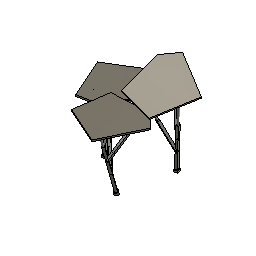
TT-3 (Autodesk Fusion 360 design; units mm, degrees)
Autodesk Fusion 360 part; units mm, degrees
sketch "Sketch1" plane through (0, 0, 0) normal (0, 1, 0) x (1, 0, 0) in component "TT-2 v5"
  line L0 (2.5, -2.5) -> (-2.5, -2.5)
  line L1 (-2.5, -2.5) -> (-2.5, 2.5)
  line L2 (-2.5, 2.5) -> (2.5, 2.5)
  line L3 (2.5, 2.5) -> (2.5, -2.5)
  constraint horizontal L0
  constraint vertical L1
  constraint horizontal L2
  constraint vertical L3
extrude "Extrude1" add sketch "Sketch1" along normal blind 2.5 makes body 1 in component "TT-2 v5"
sketch "Sketch2" plane through (0, 0, 0) normal (0, 1, 0) x (1, 0, 0) in component "TT-2 v5"
  line L0 (1.5, -1.5) -> (-1.5, -1.5)
  line L1 (-1.5, -1.5) -> (-1.5, 1.5)
  line L2 (-1.5, 1.5) -> (1.5, 1.5)
  line L3 (1.5, 1.5) -> (1.5, -1.5)
  constraint horizontal L0
  constraint vertical L1
  constraint horizontal L2
  constraint vertical L3
extrude "Extrude2" add sketch "Sketch2" along normal blind 60 separate body makes body 2 in component "TT-2 v5"
move_body "Move1" bodies 2 to x (0.939693, -0.34202, 0) y (0.34202, 0.939693, 0) z (0, 0, 1) at (-0.0905, -0.513, 0) in component "TT-2 v5"
move_body "Move2" bodies 2 to x (1, 0, 0) y (0, 1, 0) z (0, 0, 1) at (3.3727, 9.6612, 0) in component "TT-2 v5"
sphere "SpherePrimitive1" add diameter 3 placed x (0, 0, 1) y (-0.939693, 0.34202, 0) z (-0.34202, -0.939693, 0) at (3.3241, 9.1329, 0) bodies 2 in component "TT-2 v5"
sphere "SpherePrimitive2" cut diameter 3 placed x (-1, 0, 0) y (0, 0, 1) z (0, 1, 0) at (0, 2.5, 0) bodies 1 in component "TT-2 v5"
cylinder "CylinderPrimitive1" add diameter 2.5 height 40 placed x (0.883022, -0.321394, -0.34202) y (-0.321394, 0.116978, -0.939693) z (0.34202, 0.939693, 0) at (23.8453, 65.5145, 0) separate body makes body 3 in component "TT-2 v5"
sphere "SpherePrimitive3" add diameter 2.5 placed x (0, 0, -1) y (-0.939693, 0.34202, 0) z (0.34202, 0.939693, 0) at (37.5261, 103.1022, 0) bodies 3 in component "TT-2 v5"
move_body "Move3" bodies 3 2 to x (0.939693, 0.34202, 0) y (-0.34202, 0.939693, 0) z (0, 0, 1) at (23.6283, -3.8286, 0) in component "TT-2 v5"
move_body "Move4" bodies 2 3 to x (1, 0, 0) y (0, 1, 0) z (0, 0, 1) at (-23.6681, -3.196, 0) in component "TT-2 v5"
copy_body "CopyPasteBodies1" bodies 3 2 makes body 4 makes body 5 in component "TT-2 v5"
move_body "Move5" bodies 4 5 to x (1, 0, 0) y (0, 0.906308, 0.422618) z (0, -0.422618, 0.906308) at (0, 42.015, -10.6133) in component "TT-2 v5"
move_body "Move6" bodies 5 4 to x (1, 0, 0) y (0, 1, 0) z (0, 0, 1) at (0, -2.8403, 9.6134) in component "TT-2 v5"
extrude "Extrude3" cut 1 faces at (0.4157, 96.2065, 25.0427) along direction (0, -0.906308, -0.422618) blind 15 on bodies 5 bodies 5 in component "TT-2 v5"
move_body "Move7" bodies 4 to x (1, 0, 0) y (0, 1, 0) z (0, 0, 1) at (0, -26.7116, -12.4558) in component "TT-2 v5"
move_body "Move8" bodies 5 4 to x (1, 0, 0) y (0, 1, 0) z (0, 0, 1) at (0, -15.5908, 0) in component "TT-2 v5"
copy_body "CopyPasteBodies2" bodies 4 5 makes body 6 makes body 7 in component "TT-2 v5"
move_body "Move9" bodies 6 7 to x (0, 0, -1) y (0, 1, 0) z (1, 0, 0) at (-0.0791, 0, -0.06) in component "TT-2 v5"
move_body "Move10" bodies 6 to x (1, 0, 0) y (0, 1, 0) z (0, 0, 1) at (5.2397, 11.2365, 0) in component "TT-2 v5"
move_body "Move11" bodies 7 3 4 2 5 6 to x (1, 0, 0) y (0, 0.984808, -0.173648) z (0, 0.173648, 0.984808) at (0, 0.0409, 0.4679) in component "TT-2 v5"
move_body "Move12" bodies 5 4 to x (1, 0, 0) y (0, 1, 0) z (0, 0, 1) at (0, 17.3834, -3.0131) in component "TT-2 v5"
sketch "Sketch7" plane through (0, 0, 0) normal (0, 1, 0) x (1, 0, 0) in component "TT-2 v5"
  line L0 (20, -30) -> (50, 15)
  line L1 (50, 15) -> (20, 47.2574)
  line L2 (20, 47.2574) -> (-26.886, 18.4817)
  line L3 (-26.886, 18.4817) -> (-3.443, -34.2088)
  line L4 (-3.443, -34.2088) -> (20, -30)
extrude "Extrude4" add sketch "Sketch7" along normal blind 2 separate body makes body 8 in component "TT-2 v5"
move_body "Move13" bodies 8 to x (1, 0, 0) y (0, 1, 0) z (0, 0, 1) at (0, 114.7446, 0) in component "TT-2 v5"
sketch "Sketch8" plane through (0, 114.7446, 0) normal (0, -1, 0) x (1, 0, 0) in component "TT-2 v5"
  line L0 (20, 30) -> (-3.443, 34.2088)
  line L1 (-3.443, 34.2088) -> (-26.886, -18.4817)
  line L2 (-26.886, -18.4817) -> (20, -47.2574)
  line L3 (20, -47.2574) -> (50, -15)
  line L4 (50, -15) -> (20, 30)
sphere "SpherePrimitive4" cut diameter 2.5 placed x (1, 0, 0) y (0, 0, 1) z (0, -1, 0) at (-5, 114.7446, -17) bodies 8 in component "TT-2 v5"
sphere "SpherePrimitive5" cut diameter 2.5 placed x (1, 0, 0) y (0, 0, 1) z (0, -1, 0) at (3, 114.7446, 17) bodies 8 in component "TT-2 v5"
sphere "SpherePrimitive6" cut diameter 2.5 placed x (1, 0, 0) y (0, 0, 1) z (0, -1, 0) at (32.239, 114.7446, -14.3242) bodies 8 in component "TT-2 v5"
copy_body "CopyPasteBodies3" bodies 7 5 makes body 9 makes body 10 in component "TT-2 v5"
extrude "Extrude5" cut 1 faces at (19.5306, 65.7186, -10.5804) along direction (-0.422618, -0.892539, 0.157379) blind 45 on bodies 9 bodies 9 in component "TT-2 v5"
extrude "Extrude6" cut 1 faces at (-0.5843, 86.4162, 5.2019) along direction (0, -0.965926, -0.258819) blind 45 on bodies 10 bodies 10 in component "TT-2 v5"
combine "Combine1" operation cut target body 2 tool bodies 9 in component "TT-2 v5"
combine "Combine2" operation cut target body 2 tool bodies 10 in component "TT-2 v5"
copy_body "CopyPasteBodies4" bodies 7 5 makes body 11 makes body 12 in component "TT-2 v5"
combine "Combine3" operation cut target body 2 tool bodies 11 12 in component "TT-2 v5"
copy_body "Body->Comp1" bodies 1 removing the originals makes body 13 in component "MainFix"
copy_body "Body->Comp2" bodies 3 removing the originals makes body 14 in component "MainAct"
copy_body "Body->Comp3" bodies 4 removing the originals makes body 15 in component "LeftAct"
copy_body "Body->Comp4" bodies 2 removing the originals makes body 16 in component "MainBranch"
copy_body "Body->Comp5" bodies 5 removing the originals makes body 17 in component "LeftBranch"
copy_body "Body->Comp6" bodies 6 removing the originals makes body 18 in component "RightAct"
copy_body "Body->Comp7" bodies 7 removing the originals makes body 19 in component "RightBranch"
copy_body "Body->Comp8" bodies 8 removing the originals makes body 20 in component "Flat"
sketch "Sketch1 (2)" plane through (0, 0, 0) normal (0, 1, 0) x (1, 0, 0) in component "TT-2 v5 (1)"
  line L0 (2.5, -2.5) -> (-2.5, -2.5)
  line L1 (-2.5, -2.5) -> (-2.5, 2.5)
  line L2 (-2.5, 2.5) -> (2.5, 2.5)
  line L3 (2.5, 2.5) -> (2.5, -2.5)
  constraint horizontal L0
  constraint vertical L1
  constraint horizontal L2
  constraint vertical L3
extrude "Extrude1'" add sketch "Sketch1 (2)" along normal blind 2.5 separate body makes body 21 in component "TT-2 v5 (1)"
sketch "Sketch2 (2)" plane through (0, 0, 0) normal (0, 1, 0) x (1, 0, 0) in component "TT-2 v5 (1)"
  line L0 (1.5, -1.5) -> (-1.5, -1.5)
  line L1 (-1.5, -1.5) -> (-1.5, 1.5)
  line L2 (-1.5, 1.5) -> (1.5, 1.5)
  line L3 (1.5, 1.5) -> (1.5, -1.5)
  constraint horizontal L0
  constraint vertical L1
  constraint horizontal L2
  constraint vertical L3
extrude "Extrude2'" add sketch "Sketch2 (2)" along normal blind 60 separate body makes body 22 in component "TT-2 v5 (1)"
move_body "Move1'" bodies 22 to x (0.939693, -0.34202, 0) y (0.34202, 0.939693, 0) z (0, 0, 1) at (-0.0905, -0.513, 0) in component "TT-2 v5 (1)"
move_body "Move2'" bodies 22 to x (1, 0, 0) y (0, 1, 0) z (0, 0, 1) at (3.3727, 9.6612, 0) in component "TT-2 v5 (1)"
sphere "SpherePrimitive1'" add diameter 3 placed x (0, 0, 1) y (-0.939693, 0.34202, 0) z (-0.34202, -0.939693, 0) at (3.3241, 9.1329, 0) bodies 22 in component "TT-2 v5 (1)"
sphere "SpherePrimitive2'" cut diameter 3 placed x (-1, 0, 0) y (0, 0, 1) z (0, 1, 0) at (0, 2.5, 0) bodies 21 in component "TT-2 v5 (1)"
cylinder "CylinderPrimitive1'" add diameter 2.5 height 40 placed x (0.883022, -0.321394, -0.34202) y (-0.321394, 0.116978, -0.939693) z (0.34202, 0.939693, 0) at (23.8453, 65.5145, 0) separate body makes body 23 in component "TT-2 v5 (1)"
sphere "SpherePrimitive3'" add diameter 2.5 placed x (0, 0, -1) y (-0.939693, 0.34202, 0) z (0.34202, 0.939693, 0) at (37.5261, 103.1022, 0) bodies 23 in component "TT-2 v5 (1)"
move_body "Move3'" bodies 23 22 to x (0.939693, 0.34202, 0) y (-0.34202, 0.939693, 0) z (0, 0, 1) at (23.6283, -3.8286, 0) in component "TT-2 v5 (1)"
move_body "Move4'" bodies 22 23 to x (1, 0, 0) y (0, 1, 0) z (0, 0, 1) at (-23.6681, -3.196, 0) in component "TT-2 v5 (1)"
copy_body "CopyPasteBodies1'" bodies 23 22 makes body 24 makes body 25 in component "TT-2 v5 (1)"
move_body "Move5'" bodies 24 25 to x (1, 0, 0) y (0, 0.906308, 0.422618) z (0, -0.422618, 0.906308) at (0, 42.015, -10.6133) in component "TT-2 v5 (1)"
move_body "Move6'" bodies 25 24 to x (1, 0, 0) y (0, 1, 0) z (0, 0, 1) at (0, -2.8403, 9.6134) in component "TT-2 v5 (1)"
extrude "Extrude3'" cut 1 faces at (0.4157, 96.2065, 25.0427) along direction (0, -0.906308, -0.422618) blind 15 on bodies 25 bodies 25 in component "TT-2 v5 (1)"
move_body "Move7'" bodies 24 to x (1, 0, 0) y (0, 1, 0) z (0, 0, 1) at (0, -26.7116, -12.4558) in component "TT-2 v5 (1)"
move_body "Move8'" bodies 25 24 to x (1, 0, 0) y (0, 1, 0) z (0, 0, 1) at (0, -15.5908, 0) in component "TT-2 v5 (1)"
copy_body "CopyPasteBodies2'" bodies 24 25 makes body 26 makes body 27 in component "TT-2 v5 (1)"
move_body "Move9'" bodies 26 27 to x (0, 0, -1) y (0, 1, 0) z (1, 0, 0) at (-0.0791, 0, -0.06) in component "TT-2 v5 (1)"
move_body "Move10'" bodies 26 to x (1, 0, 0) y (0, 1, 0) z (0, 0, 1) at (5.2397, 11.2365, 0) in component "TT-2 v5 (1)"
move_body "Move11'" bodies 27 23 24 22 25 26 to x (1, 0, 0) y (0, 0.984808, -0.173648) z (0, 0.173648, 0.984808) at (0, 0.0409, 0.4679) in component "TT-2 v5 (1)"
move_body "Move12'" bodies 25 24 to x (1, 0, 0) y (0, 1, 0) z (0, 0, 1) at (0, 17.3834, -3.0131) in component "TT-2 v5 (1)"
sketch "Sketch7 (2)" plane through (0, 0, 0) normal (0, 1, 0) x (1, 0, 0) in component "TT-2 v5 (1)"
  line L0 (20, -30) -> (50, 15)
  line L1 (50, 15) -> (20, 47.2574)
  line L2 (20, 47.2574) -> (-26.886, 18.4817)
  line L3 (-26.886, 18.4817) -> (-3.443, -34.2088)
  line L4 (-3.443, -34.2088) -> (20, -30)
extrude "Extrude4'" add sketch "Sketch7 (2)" along normal blind 2 separate body makes body 28 in component "TT-2 v5 (1)"
move_body "Move13'" bodies 28 to x (1, 0, 0) y (0, 1, 0) z (0, 0, 1) at (0, 114.7446, 0) in component "TT-2 v5 (1)"
sketch "Sketch8 (2)" plane through (0, 114.7446, 0) normal (0, -1, 0) x (1, 0, 0) in component "TT-2 v5 (1)"
  line L0 (20, 30) -> (-3.443, 34.2088)
  line L1 (-3.443, 34.2088) -> (-26.886, -18.4817)
  line L2 (-26.886, -18.4817) -> (20, -47.2574)
  line L3 (20, -47.2574) -> (50, -15)
  line L4 (50, -15) -> (20, 30)
sphere "SpherePrimitive4'" cut diameter 2.5 placed x (1, 0, 0) y (0, 0, 1) z (0, -1, 0) at (-5, 114.7446, -17) bodies 28 in component "TT-2 v5 (1)"
sphere "SpherePrimitive5'" cut diameter 2.5 placed x (1, 0, 0) y (0, 0, 1) z (0, -1, 0) at (3, 114.7446, 17) bodies 28 in component "TT-2 v5 (1)"
sphere "SpherePrimitive6'" cut diameter 2.5 placed x (1, 0, 0) y (0, 0, 1) z (0, -1, 0) at (32.239, 114.7446, -14.3242) bodies 28 in component "TT-2 v5 (1)"
copy_body "CopyPasteBodies3'" bodies 27 25 makes body 29 makes body 30 in component "TT-2 v5 (1)"
extrude "Extrude5'" cut 1 faces at (19.5306, 65.7186, -10.5804) along direction (-0.422618, -0.892539, 0.157379) blind 45 on bodies 29 bodies 29 in component "TT-2 v5 (1)"
extrude "Extrude6'" cut 1 faces at (-0.5843, 86.4162, 5.2019) along direction (0, -0.965926, -0.258819) blind 45 on bodies 30 bodies 30 in component "TT-2 v5 (1)"
combine "Combine1'" operation cut target body 22 tool bodies 29 in component "TT-2 v5 (1)"
combine "Combine2'" operation cut target body 22 tool bodies 30 in component "TT-2 v5 (1)"
copy_body "CopyPasteBodies4'" bodies 27 25 makes body 31 makes body 32 in component "TT-2 v5 (1)"
combine "Combine3'" operation cut target body 22 tool bodies 31 32 in component "TT-2 v5 (1)"
copy_body "Body->Comp1'" bodies 21 removing the originals makes body 33 in component "MainFix (1)"
copy_body "Body->Comp2'" bodies 23 removing the originals makes body 34 in component "MainAct (1)"
copy_body "Body->Comp3'" bodies 24 removing the originals makes body 35 in component "LeftAct (1)"
copy_body "Body->Comp4'" bodies 22 removing the originals makes body 36 in component "MainBranch (1)"
copy_body "Body->Comp5'" bodies 25 removing the originals makes body 37 in component "LeftBranch (1)"
copy_body "Body->Comp6'" bodies 26 removing the originals makes body 38 in component "RightAct (1)"
copy_body "Body->Comp7'" bodies 27 removing the originals makes body 39 in component "RightBranch (1)"
copy_body "Body->Comp8'" bodies 28 removing the originals makes body 40 in component "Flat (1)"
sketch "Sketch1 (3)" plane through (0, 0, 0) normal (0, 1, 0) x (1, 0, 0) in component "TT-2 v5 (2)"
  line L0 (2.5, -2.5) -> (-2.5, -2.5)
  line L1 (-2.5, -2.5) -> (-2.5, 2.5)
  line L2 (-2.5, 2.5) -> (2.5, 2.5)
  line L3 (2.5, 2.5) -> (2.5, -2.5)
  constraint horizontal L0
  constraint vertical L1
  constraint horizontal L2
  constraint vertical L3
extrude "Extrude1''" add sketch "Sketch1 (3)" along normal blind 2.5 separate body makes body 41 in component "TT-2 v5 (2)"
sketch "Sketch2 (3)" plane through (0, 0, 0) normal (0, 1, 0) x (1, 0, 0) in component "TT-2 v5 (2)"
  line L0 (1.5, -1.5) -> (-1.5, -1.5)
  line L1 (-1.5, -1.5) -> (-1.5, 1.5)
  line L2 (-1.5, 1.5) -> (1.5, 1.5)
  line L3 (1.5, 1.5) -> (1.5, -1.5)
  constraint horizontal L0
  constraint vertical L1
  constraint horizontal L2
  constraint vertical L3
extrude "Extrude2''" add sketch "Sketch2 (3)" along normal blind 60 separate body makes body 42 in component "TT-2 v5 (2)"
move_body "Move1''" bodies 42 to x (0.939693, -0.34202, 0) y (0.34202, 0.939693, 0) z (0, 0, 1) at (-0.0905, -0.513, 0) in component "TT-2 v5 (2)"
move_body "Move2''" bodies 42 to x (1, 0, 0) y (0, 1, 0) z (0, 0, 1) at (3.3727, 9.6612, 0) in component "TT-2 v5 (2)"
sphere "SpherePrimitive1''" add diameter 3 placed x (0, 0, 1) y (-0.939693, 0.34202, 0) z (-0.34202, -0.939693, 0) at (3.3241, 9.1329, 0) bodies 42 in component "TT-2 v5 (2)"
sphere "SpherePrimitive2''" cut diameter 3 placed x (-1, 0, 0) y (0, 0, 1) z (0, 1, 0) at (0, 2.5, 0) bodies 41 in component "TT-2 v5 (2)"
cylinder "CylinderPrimitive1''" add diameter 2.5 height 40 placed x (0.883022, -0.321394, -0.34202) y (-0.321394, 0.116978, -0.939693) z (0.34202, 0.939693, 0) at (23.8453, 65.5145, 0) separate body makes body 43 in component "TT-2 v5 (2)"
sphere "SpherePrimitive3''" add diameter 2.5 placed x (0, 0, -1) y (-0.939693, 0.34202, 0) z (0.34202, 0.939693, 0) at (37.5261, 103.1022, 0) bodies 43 in component "TT-2 v5 (2)"
move_body "Move3''" bodies 43 42 to x (0.939693, 0.34202, 0) y (-0.34202, 0.939693, 0) z (0, 0, 1) at (23.6283, -3.8286, 0) in component "TT-2 v5 (2)"
move_body "Move4''" bodies 42 43 to x (1, 0, 0) y (0, 1, 0) z (0, 0, 1) at (-23.6681, -3.196, 0) in component "TT-2 v5 (2)"
copy_body "CopyPasteBodies1''" bodies 43 42 makes body 44 makes body 45 in component "TT-2 v5 (2)"
move_body "Move5''" bodies 44 45 to x (1, 0, 0) y (0, 0.906308, 0.422618) z (0, -0.422618, 0.906308) at (0, 42.015, -10.6133) in component "TT-2 v5 (2)"
move_body "Move6''" bodies 45 44 to x (1, 0, 0) y (0, 1, 0) z (0, 0, 1) at (0, -2.8403, 9.6134) in component "TT-2 v5 (2)"
extrude "Extrude3''" cut 1 faces at (0.4157, 96.2065, 25.0427) along direction (0, -0.906308, -0.422618) blind 15 on bodies 45 bodies 45 in component "TT-2 v5 (2)"
move_body "Move7''" bodies 44 to x (1, 0, 0) y (0, 1, 0) z (0, 0, 1) at (0, -26.7116, -12.4558) in component "TT-2 v5 (2)"
move_body "Move8''" bodies 45 44 to x (1, 0, 0) y (0, 1, 0) z (0, 0, 1) at (0, -15.5908, 0) in component "TT-2 v5 (2)"
copy_body "CopyPasteBodies2''" bodies 44 45 makes body 46 makes body 47 in component "TT-2 v5 (2)"
move_body "Move9''" bodies 46 47 to x (0, 0, -1) y (0, 1, 0) z (1, 0, 0) at (-0.0791, 0, -0.06) in component "TT-2 v5 (2)"
move_body "Move10''" bodies 46 to x (1, 0, 0) y (0, 1, 0) z (0, 0, 1) at (5.2397, 11.2365, 0) in component "TT-2 v5 (2)"
move_body "Move11''" bodies 47 43 44 42 45 46 to x (1, 0, 0) y (0, 0.984808, -0.173648) z (0, 0.173648, 0.984808) at (0, 0.0409, 0.4679) in component "TT-2 v5 (2)"
move_body "Move12''" bodies 45 44 to x (1, 0, 0) y (0, 1, 0) z (0, 0, 1) at (0, 17.3834, -3.0131) in component "TT-2 v5 (2)"
sketch "Sketch7 (3)" plane through (0, 0, 0) normal (0, 1, 0) x (1, 0, 0) in component "TT-2 v5 (2)"
  line L0 (20, -30) -> (50, 15)
  line L1 (50, 15) -> (20, 47.2574)
  line L2 (20, 47.2574) -> (-26.886, 18.4817)
  line L3 (-26.886, 18.4817) -> (-3.443, -34.2088)
  line L4 (-3.443, -34.2088) -> (20, -30)
extrude "Extrude4''" add sketch "Sketch7 (3)" along normal blind 2 separate body makes body 48 in component "TT-2 v5 (2)"
move_body "Move13''" bodies 48 to x (1, 0, 0) y (0, 1, 0) z (0, 0, 1) at (0, 114.7446, 0) in component "TT-2 v5 (2)"
sketch "Sketch8 (3)" plane through (0, 114.7446, 0) normal (0, -1, 0) x (1, 0, 0) in component "TT-2 v5 (2)"
  line L0 (20, 30) -> (-3.443, 34.2088)
  line L1 (-3.443, 34.2088) -> (-26.886, -18.4817)
  line L2 (-26.886, -18.4817) -> (20, -47.2574)
  line L3 (20, -47.2574) -> (50, -15)
  line L4 (50, -15) -> (20, 30)
sphere "SpherePrimitive4''" cut diameter 2.5 placed x (1, 0, 0) y (0, 0, 1) z (0, -1, 0) at (-5, 114.7446, -17) bodies 48 in component "TT-2 v5 (2)"
sphere "SpherePrimitive5''" cut diameter 2.5 placed x (1, 0, 0) y (0, 0, 1) z (0, -1, 0) at (3, 114.7446, 17) bodies 48 in component "TT-2 v5 (2)"
sphere "SpherePrimitive6''" cut diameter 2.5 placed x (1, 0, 0) y (0, 0, 1) z (0, -1, 0) at (32.239, 114.7446, -14.3242) bodies 48 in component "TT-2 v5 (2)"
copy_body "CopyPasteBodies3''" bodies 47 45 makes body 49 makes body 50 in component "TT-2 v5 (2)"
extrude "Extrude5''" cut 1 faces at (19.5306, 65.7186, -10.5804) along direction (-0.422618, -0.892539, 0.157379) blind 45 on bodies 49 bodies 49 in component "TT-2 v5 (2)"
extrude "Extrude6''" cut 1 faces at (-0.5843, 86.4162, 5.2019) along direction (0, -0.965926, -0.258819) blind 45 on bodies 50 bodies 50 in component "TT-2 v5 (2)"
combine "Combine1''" operation cut target body 42 tool bodies 49 in component "TT-2 v5 (2)"
combine "Combine2''" operation cut target body 42 tool bodies 50 in component "TT-2 v5 (2)"
copy_body "CopyPasteBodies4''" bodies 47 45 makes body 51 makes body 52 in component "TT-2 v5 (2)"
combine "Combine3''" operation cut target body 42 tool bodies 51 52 in component "TT-2 v5 (2)"
copy_body "Body->Comp1''" bodies 41 removing the originals makes body 53 in component "MainFix (2)"
copy_body "Body->Comp2''" bodies 43 removing the originals makes body 54 in component "MainAct (2)"
copy_body "Body->Comp3''" bodies 44 removing the originals makes body 55 in component "LeftAct (2)"
copy_body "Body->Comp4''" bodies 42 removing the originals makes body 56 in component "MainBranch (2)"
copy_body "Body->Comp5''" bodies 45 removing the originals makes body 57 in component "LeftBranch (2)"
copy_body "Body->Comp6''" bodies 46 removing the originals makes body 58 in component "RightAct (2)"
copy_body "Body->Comp7''" bodies 47 removing the originals makes body 59 in component "RightBranch (2)"
copy_body "Body->Comp8''" bodies 48 removing the originals makes body 60 in component "Flat (2)"
component "TT-2 v5" placed x (1, 0, 0) y (0, 1, 0) z (0, 0, 1) at (0, 0, 0)
component "TT-2 v5 (1)" placed x (-0.965926, 0, 0.258819) y (0, 1, 0) z (-0.258819, 0, -0.965926) at (65.1368, 0, -31.6941)
component "TT-2 v5 (2)" placed x (-0.793623, 0, -0.60841) y (0, 1, 0) z (0.60841, 0, -0.793623) at (50.4677, 0, 35.3299)
component "MainFix" placed x (1, 0, 0) y (0, 1, 0) z (0, 0, 1) at (0, 0, 0) in component "TT-2 v5"
component "MainAct" placed x (0.988019, 0.153888, 0.011707) y (-0.151963, 0.983285, -0.100286) z (-0.026944, 0.097305, 0.99489) at (3.0787, -17.6984, 5.278) in component "TT-2 v5"
component "LeftAct" placed x (0.988178, -0.114692, 0.101738) y (0.083546, 0.959254, 0.269912) z (-0.128549, -0.258222, 0.957495) at (-11.6629, -23.6616, -29.0003) in component "TT-2 v5"
component "MainBranch" placed x (0.988019, 0.153888, 0.011707) y (-0.151963, 0.983285, -0.100286) z (-0.026944, 0.097305, 0.99489) at (0.4488, -0.1433, 0.2707) in component "TT-2 v5"
component "LeftBranch" placed x (0.988178, -0.114692, 0.101738) y (0.083546, 0.959254, 0.269912) z (-0.128549, -0.258222, 0.957495) at (-10.4005, -1.5818, -15.9325) in component "TT-2 v5"
component "RightAct" placed x (0.972319, -0.069652, -0.223035) y (0.081853, 0.995586, 0.045925) z (0.218851, -0.062909, 0.973728) at (-13.1743, -17.7837, 0.4548) in component "TT-2 v5"
component "RightBranch" placed x (0.972319, -0.069652, -0.223035) y (0.081853, 0.995586, 0.045925) z (0.218851, -0.062909, 0.973728) at (-4.5511, -1.098, -3.5544) in component "TT-2 v5"
component "Flat" placed x (1, 0, 0) y (0, 1, 0) z (0, 0, 1) at (-6.8676, -34.6546, -5.1449) in component "TT-2 v5"
component "MainFix (1)" placed x (1, 0, 0) y (0, 1, 0) z (0, 0, 1) at (0, 0, 0) in component "TT-2 v5 (1)"
component "MainAct (1)" placed x (0.9909, 0.114896, 0.070121) y (-0.117343, 0.992581, 0.031835) z (-0.065943, -0.039774, 0.99703) at (0.3801, -0.8237, 0.0073) in component "TT-2 v5 (1)"
component "LeftAct (1)" placed x (-0.118508, -0.23576, 0.964558) y (0.447944, 0.854247, 0.263833) z (-0.886173, 0.463335, 0.004372) at (-29.6383, 9.6407, -16.8615) in component "TT-2 v5 (1)"
component "MainBranch (1)" placed x (0.9909, 0.114896, 0.070121) y (-0.117343, 0.992581, 0.031835) z (-0.065943, -0.039774, 0.99703) at (0.3556, -0.1699, -0.083) in component "TT-2 v5 (1)"
component "LeftBranch (1)" placed x (-0.118508, -0.23576, 0.964558) y (0.447944, 0.854247, 0.263833) z (-0.886173, 0.463335, 0.004372) at (-29.723, 9.2609, -16.9186) in component "TT-2 v5 (1)"
component "RightAct (1)" placed x (0.923021, 0.229892, 0.308517) y (-0.133967, 0.943716, -0.302411) z (-0.360674, 0.2378, 0.901868) at (-0.4404, 2.1978, 8.1405) in component "TT-2 v5 (1)"
component "RightBranch (1)" placed x (0.923021, 0.229892, 0.308517) y (-0.133967, 0.943716, -0.302411) z (-0.360674, 0.2378, 0.901868) at (-0.4136, 2.2076, 8.0947) in component "TT-2 v5 (1)"
component "Flat (1)" placed x (0.916563, -0.021172, -0.39933) y (-0.096266, 0.957549, -0.271722) z (0.388131, 0.287492, 0.875616) at (11.8405, -4.8051, 29.9797) in component "TT-2 v5 (1)"
component "MainFix (2)" placed x (1, 0, 0) y (0, 1, 0) z (0, 0, 1) at (0, 0, 0) in component "TT-2 v5 (2)"
component "MainAct (2)" placed x (0.989237, 0.127632, 0.071552) y (-0.124231, 0.990986, -0.050136) z (-0.077306, 0.040708, 0.996176) at (2.9999, -23.9191, 5.5851) in component "TT-2 v5 (2)"
component "LeftAct (2)" placed x (0.815945, -0.214594, 0.536827) y (-0.010264, 0.923035, 0.38458) z (-0.578038, -0.319306, 0.750943) at (-4.2908, -18.7878, -33.6197) in component "TT-2 v5 (2)"
component "MainBranch (2)" placed x (0.989237, 0.127632, 0.071552) y (-0.124231, 0.990986, -0.050136) z (-0.077306, 0.040708, 0.996176) at (0.3741, -0.1651, 0.1379) in component "TT-2 v5 (2)"
component "LeftBranch (2)" placed x (0.815945, -0.214594, 0.536827) y (-0.010264, 0.923035, 0.38458) z (-0.578038, -0.319306, 0.750943) at (-8.0114, 0.2544, -20.2696) in component "TT-2 v5 (2)"
component "RightAct (2)" placed x (-0.08378, 0.474005, 0.876527) y (0.3797, 0.828445, -0.411711) z (-0.921308, 0.298324, -0.249387) at (-24.913, -12.7473, 3.4438) in component "TT-2 v5 (2)"
component "RightBranch (2)" placed x (-0.08378, 0.474005, 0.876527) y (0.3797, 0.828445, -0.411711) z (-0.921308, 0.298324, -0.249387) at (-15.9329, 5.0351, 4.2997) in component "TT-2 v5 (2)"
component "Flat (2)" placed x (0.937756, 0.146692, 0.314793) y (-0.10576, 0.983986, -0.143477) z (-0.330799, 0.101254, 0.938253) at (2.9344, -34.8202, 17.1988) in component "TT-2 v5 (2)"
named bodies: "MainFix", "MainBranch", "MainAct", "LeftAct", "LeftBranch", "MainAct (1)", "MainBranch (1)", "RightAct", "RightBranch", "Flat", "RightBranch (1)", "LeftBranch (1)"
